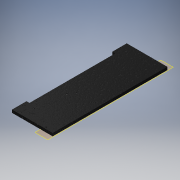
# Autodesk Inventor part: fronts
Saved by Autodesk Inventor 2018 (Build 220112000, 112)
## iProperties
Created: 2017-10-09
Part Number: fronts
Material: Generic
Document SubType Name: Modeling
Designer: HP
Density: 1 g/cm^3
Appearance: Fine Textured - Black
Author: HP
Autodesk Inventor part; units mm, degrees
ref_plane "YZ Plane" through (0, 0, 0) normal (1, 0, 0) x (0, 1, 0)
ref_plane "XZ Plane" through (0, 0, 0) normal (0, 1, 0) x (-1, 0, 0)
ref_plane "XY Plane" through (0, 0, 0) normal (0, 0, 1) x (1, 0, 0)
ref_plane "Work Plane1" through (0, 0, -0.5) normal (0, 0, 1) x (1, 0, 0)
sketch "Sketch1" plane through (0, 0, -0.5) normal (0, 0, 1) x (1, 0, 0)
  line L0 (0, 197) -> (0, 0) construction
  line L1 (0, 197) -> (-20, 197) construction
  line L2 (-20, 0) -> (-20, 197) construction
  line L3 (0, 0) -> (-20, 0) construction
  line L4 (0, -0.5) -> (-70, -0.5) construction
  line L5 (-70, -0.5) -> (-70, -5.5) construction
  line L6 (0, -5.5) -> (-70, -5.5) construction
  line L7 (0, -0.5) -> (0, -5.5) construction
  line L8 (-70, 197.5) -> (0, 197.5) construction
  line L9 (0, 197.5) -> (0, 202.5) construction
  line L10 (-70, 202.5) -> (0, 202.5) construction
  line L11 (-70, 197.5) -> (-70, 202.5) construction
  line L12 (0, -0.4) -> (0, 197.4)
  line L13 (0, -0.4) -> (-70, -0.4)
  line L14 (-70, -0.4) -> (-70, 24.5)
  line L15 (-70, 24.5) -> (-64.9, 24.5)
  line L16 (-64.9, 24.5) -> (-64.9, 172.5)
  line L17 (-64.9, 172.5) -> (-70, 172.5)
  line L18 (-70, 172.5) -> (-70, 197.4)
  line L19 (-70, 197.4) -> (0, 197.4)
  line L20 (-64.9, -0.5) -> (-64.9, -5.5) construction
  dimension "d1" = 0.1
  dimension "d2" = 0.1
  dimension "d3" = 24.9
  dimension "d4" = 24.9
  constraints: 16 end point, 6 perpendicular, 4 collinear, 1 point on line, 1 vertical
  measures "d1" distance from line of L12.start L4
  measures "d2" distance from line of L12.end L8
  measures "d3" distance between parallel lines of L15 L13
  measures "d4" distance between parallel lines of L17 L19
extrude "Extrusion1" add sketch "Sketch1" along normal blind 5
equation "\"d1\" = ABS_tolerance"
equation "\"d2\" = ABS_tolerance"
equation "\"d4\" = d3"
equation "\"d5\" = plate_thickness"
equation "\"plate_thickness\" = 5"
equation "\"basic_plate_offset\" = 0.5"
equation "\"ABS_tolerance\" = 0.1"
equation "\"laser_cutter_thickness\" = 0.1"
body "Solid1"
